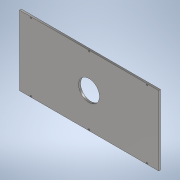
# Autodesk Inventor part: base-inferior
Saved by Autodesk Inventor 2021 (Build 250183000, 183)
## iProperties
Created: 2023-11-09
Part Number: base-inferior
Material: Genérico
Document SubType Name: Modeling
Designer: Vinicius
Density: 1 g/cm^3
Appearance: Padrão
Author: Vinicius
Autodesk Inventor part; units mm, degrees
ref_plane "YZ Plane" through (0, 0, 0) normal (1, 0, 0) x (0, 1, 0)
ref_plane "XZ Plane" through (0, 0, 0) normal (0, 1, 0) x (-1, 0, 0)
ref_plane "XY Plane" through (0, 0, 0) normal (0, 0, 1) x (1, 0, 0)
sketch "Esboço1" plane through (0, 0, 0) normal (0, 0, 1) x (1, 0, 0)
  line L0 (-300, -150) -> (300, -150)
  line L1 (300, -150) -> (300, 150)
  line L2 (300, 150) -> (-300, 150)
  line L3 (-300, 150) -> (-300, -150)
  line L4 (-300, -150) -> (300, 150) construction
  line L5 (300, -150) -> (-300, 150) construction
  circle A0 centre (0, 0) radius 45
  dimension "d0" = 600
  dimension "d1" = 300
  dimension "d2" = 90
  constraints: 12 end point, 2 midpoint, 2 parallel, 1 centre point, 1 coincident, 1 horizontal, 1 perpendicular
  measures "d0" distance of L1.end L2.end
  measures "d1" distance of L2.end L0.start
  measures "d2" diameter of A0
extrude "Extrusão1" add sketch "Esboço1" along normal blind 8
sketch "Esboço2" plane through (0, 0, 8) normal (0, 0, 1) x (1, 0, 0)
  line L0 (-250, -146) -> (250, 146) construction
  line L1 (250, -146) -> (-250, 146) construction
  circle A0 centre (-250, 146) radius 2
  circle A1 centre (0, 146) radius 2
  circle A2 centre (250, 146) radius 2
  circle A3 centre (250, -146) radius 2
  circle A4 centre (0, -146) radius 2
  circle A5 centre (-250, -146) radius 2
  point P0 (0, 0)
  dimension "d5" = 292
  dimension "d7" = 4
  dimension "d8" = 4
  dimension "d9" = 4
  dimension "d10" = 4
  dimension "d11" = 4
  dimension "d12" = 4
  constraints: 6 centre point, 4 end point, 2 midpoint, 1 coincident
  measures "d5" distance of L1.start L0.end
  measures "d7" diameter of A0
  measures "d8" diameter of A1
  measures "d9" diameter of A2
  measures "d10" diameter of A3
  measures "d11" diameter of A4
  measures "d12" diameter of A5
extrude "Extrusão2" cut sketch "Esboço2" against normal blind 10
chamfer "Chanfro1" distance 1 angle 45 6 edges at (-252, 146, 8) (-2, 146, 8) (248, 146, 8) (248, -146, 8) (-2, -146, 8) (-252, -146, 8)
